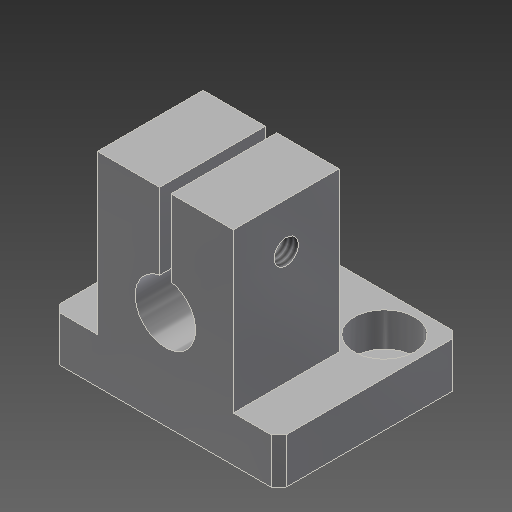
# Autodesk Inventor part: 06
Saved by Autodesk Inventor 2021.1 (Build 251245010, 245A)
## iProperties
Created: 2010-03-11
Part Number: 06
Document SubType Name: Modeling
Density: 1 g/cm^3
Material: SUS303
Appearance: 鋼
Title: ブロック
Autodesk Inventor part; units mm, degrees
note: some values were not read from the file. Chosen so that the rebuilt part matches the saved one: direction of "穴3"; direction of "穴4".
ref_plane "YZ Plane" through (0, 0, 0) normal (1, 0, 0) x (0, 1, 0)
ref_plane "XZ Plane" through (0, 0, 0) normal (0, 1, 0) x (-1, 0, 0)
ref_plane "XY Plane" through (0, 0, 0) normal (0, 0, 1) x (1, 0, 0)
sketch "スケッチ1" plane through (0, 0, 0) normal (0, 0, 1) x (1, 0, 0)
  line L0 (-9, 21) -> (9, 21)
  line L1 (9, 21) -> (9, 0)
  line L2 (9, 0) -> (-9, 0)
  line L3 (-9, 0) -> (-9, 21)
  point P0 (0, 0)
  point P1 (0, 0)
  dimension "d0" = 18
  dimension "d1" = 21
  constraints: 8 end point, 2 parallel, 1 coincident, 1 horizontal, 1 midpoint, 1 perpendicular
  measures "d0" distance of L1.end L2.end
  measures "d1" distance of L2.end L0.start
extrude "押し出し1" add sketch "スケッチ1" along normal blind 14
sketch "スケッチ3" plane through (0, 0, 14) normal (0, 0, 1) x (1, 0, 0)
  line L0 (-9, 21) -> (9, 21) projected
  point P0 (0, 0)
  point P1 (0, 7)
  point P2 (0, 21)
  dimension "d41" = 14
  constraints: 1 midpoint, 1 vertical alignment
  measures "d41" distance from line of point (0, 7) L0
hole "穴2" at (0, 7, 14) direction (0, 0, -1) diameter 8 end through all
sketch "スケッチ4" plane through (-9, 21, 0) normal (0, 1, 0) x (1, 0, 0)
  line L0 (0, -14) -> (18, -14) projected
  line L1 (0, 0) -> (18, 0) projected
  line L2 (8.25, 0) -> (9.75, 0)
  line L3 (9.75, 0) -> (9.75, -14)
  line L4 (9.75, -14) -> (8.25, -14)
  line L5 (8.25, -14) -> (8.25, 0)
  point P0 (9, 0)
  point P1 (9, 0)
  point P2 (9, 0)
  dimension "d21" = 1.5
  constraints: 8 end point, 2 midpoint, 2 parallel, 2 point on line, 1 coincident, 1 horizontal, 1 perpendicular
  measures "d21" distance of L3.end L4.end
extrude "押し出し2" cut sketch "スケッチ4" against normal up to surface
sketch "スケッチ5" plane through (-9, 0, 0) normal (-1, 0, 0) x (0, 0, 1)
  line L0 (0, 21) -> (14, 21) projected
  point P0 (7, 15)
  point P1 (7, 21)
  dimension "d42" = 6
  constraints: 1 midpoint, 1 vertical alignment
  measures "d42" distance from line of point (7, 15) L0
hole "穴3" at (-9, 15, 7) direction (1, 0, 0) diameter 4.5 end up to surface counterbore diameter 8 counterbore depth 4.5
sketch "スケッチ6" plane through (9, 0, 0) normal (1, 0, 0) x (0, 0, -1)
  circle A0 centre (-7, 15) radius 2.25 projected
hole "穴4" at (9, 15, 7) direction (-1, 0, 0) diameter 3.242 end up to surface thread size "M4x0.7" class "6H" standard "ANSI Metric M Profile"
sketch "スケッチ9" plane through (-9, 0, 0) normal (0, -1, 0) x (1, 0, 0)
  line L0 (18, 14) -> (0, 14) projected
  line L1 (18, 0) -> (0, 0) projected
  line L2 (-6, 14) -> (24, 14)
  line L3 (24, 14) -> (24, -10)
  line L4 (24, -10) -> (-6, -10)
  line L5 (-6, -10) -> (-6, 14)
  point P0 (9, -10)
  point P1 (9, 0)
  dimension "d46" = 30
  dimension "d47" = 24
  constraints: 8 end point, 2 midpoint, 2 parallel, 1 collinear, 1 horizontal, 1 perpendicular, 1 vertical alignment
  measures "d46" distance of L3.end L4.end
  measures "d47" distance of L4.end L2.start
extrude "押し出し5" add sketch "スケッチ9" along normal blind 6
sketch "スケッチ10" plane through (-9, 0, 0) normal (0, 1, 0) x (1, 0, 0)
  line L0 (24, 10) -> (-6, 10) projected
  point P0 (9, 0)
  point P1 (-1, 5)
  point P2 (19, 5)
  dimension "d50" = 10
  dimension "d51" = 10
  dimension "d52" = 5
  constraints: 1 horizontal alignment
  measures "d50" horizontal distance of point (-1, 5) point (9, 0)
  measures "d51" horizontal distance of point (19, 5) point (9, 0)
  measures "d52" distance from line of point (-1, 5) L0
hole "穴5" at (-10, 0, -5) at (10, 0, -5) direction (0, -1, 0) diameter 4.5 end through all counterbore diameter 8 counterbore depth 4.5
chamfer "面取り1" distance 1 angle 45 4 edges at (15, -3, 14) (-15, -3, 14) (-15, -3, -10) (15, -3, -10)
equation "\"d51\" = d50"
